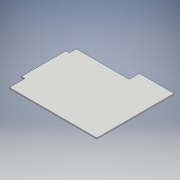
# Autodesk Inventor part: 泥除け1
Saved by Autodesk Inventor 2018 (Build 220112000, 112)
## iProperties
Created: 2017-10-08
Part Number: 泥除け1
Material: 一般
Document SubType Name: Modeling
Designer: mura5
Density: 1 g/cm^3
Appearance: 既定
Author: mura5
Autodesk Inventor part; units mm, degrees
ref_plane "YZ Plane" through (0, 0, 0) normal (1, 0, 0) x (0, 1, 0)
ref_plane "XZ Plane" through (0, 0, 0) normal (0, 1, 0) x (-1, 0, 0)
ref_plane "XY Plane" through (0, 0, 0) normal (0, 0, 1) x (1, 0, 0)
sketch "スケッチ1" plane through (0, 0, 0) normal (0, 0, 1) x (1, 0, 0)
  line L0 (-67.3, -150) -> (67.3, -150)
  line L1 (67.3, -150) -> (67.3, 150)
  line L2 (67.3, 150) -> (-67.3, 150)
  line L3 (-67.3, 150) -> (-67.3, 110)
  line L4 (-67.3, -150) -> (67.3, 150) construction
  line L5 (67.3, -150) -> (-67.3, 150) construction
  line L6 (-67.3, -150) -> (-272.7, -150)
  line L7 (-272.7, 110) -> (-67.3, 110)
  line L8 (-272.7, 82.8) -> (-286.3, 82.8)
  line L9 (-286.3, 82.8) -> (-286.3, -90)
  line L10 (-286.3, -90) -> (-272.7, -90)
  line L11 (-272.7, -150) -> (-272.7, -90)
  line L12 (-272.7, 82.8) -> (-272.7, 110)
  point P0 (0, 0)
  dimension "d0" = 134.6
  dimension "d1" = 300
  dimension "d5" = 40
  dimension "d6" = 27.2
  dimension "d8" = 13.6
  dimension "d9" = 200
  dimension "d10" = 340
  constraints: 26 end point, 4 parallel, 4 perpendicular, 3 horizontal, 2 midpoint
  measures "d0" distance of L1.end L2.end
  measures "d1" distance of L0.end L1.end
  measures "d5" distance between parallel lines of L7 L2
  measures "d6" distance between parallel lines of L8 L7
  measures "d8" distance of L9.end L10.end
  measures "d9" distance between parallel lines of L10 L7
  measures "d10" distance between parallel lines of L12 L1
extrude "押し出し1" add sketch "スケッチ1" along normal blind 4
